Autodesk Inventor part; units mm, degrees
(part 2 of 2)
  spline S48 degree 3 poles (14.8423, 75.2854) (14.8523, 75.2852) (14.8732, 75.2847) (14.9051, 75.2815) (14.9386, 75.2762) (14.9736, 75.2689) (15.0103, 75.2594) (15.0484, 75.248) (15.0882, 75.2343) (15.115, 75.224) (15.1287, 75.2187) knots 0 0 0 0 0.102203 0.211023 0.3251 0.446502 0.573788 0.708901 0.850358 1 1 1 1
  line L109 (11.6821, 74.5687) -> (11.0654, 75.8687)
  line L110 (11.0654, 75.8687) -> (11.0487, 75.8687)
  line L111 (11.0487, 75.8687) -> (10.4487, 74.5687)
  line L112 (10.4487, 74.5687) -> (10.5756, 74.5687)
  line L113 (10.5756, 74.5687) -> (10.7677, 74.9854)
  line L114 (10.7677, 74.9854) -> (11.3571, 74.9854)
  line L115 (11.3571, 74.9854) -> (11.5547, 74.5687)
  line L116 (11.5547, 74.5687) -> (11.6821, 74.5687)
  spline S49 degree 3 poles (10.1721, 75.2263) (10.1715, 75.2497) (10.1703, 75.2957) (10.1607, 75.3632) (10.1452, 75.4279) (10.1231, 75.4896) (10.0951, 75.5487) (10.0606, 75.6047) (10.0198, 75.658) (9.9732, 75.7078) (9.9221, 75.7533) (9.8674, 75.7934) (9.8092, 75.8267) (9.7481, 75.8546) (9.6837, 75.876) (9.616, 75.891) (9.5453, 75.9003) (9.4971, 75.9015) (9.4726, 75.9021) knots 0 0 0 0 0.064558 0.127014 0.187955 0.248014 0.307748 0.368235 0.42947 0.492743 0.556258 0.618217 0.679655 0.741246 0.803415 0.866815 0.932328 1 1 1 1
  spline S50 degree 3 poles (9.4726, 75.9021) (9.4576, 75.9019) (9.4281, 75.9015) (9.3843, 75.8981) (9.3418, 75.8923) (9.3003, 75.8845) (9.2598, 75.8747) (9.2205, 75.8621) (9.1822, 75.8476) (9.1451, 75.8309) (9.1095, 75.8121) (9.0753, 75.7915) (9.0428, 75.7691) (9.0118, 75.7451) (8.9828, 75.719) (8.955, 75.6914) (8.9292, 75.6616) (8.9134, 75.6407) (8.9054, 75.6302) knots 0 0 0 0 0.068548 0.135683 0.201215 0.265682 0.329267 0.392395 0.45507 0.517127 0.57879 0.63974 0.700192 0.759806 0.819628 0.879355 0.939512 1 1 1 1
  line L117 (8.9054, 75.6302) -> (9.0075, 75.5521)
  spline S51 degree 3 poles (9.0075, 75.5521) (9.0148, 75.5607) (9.0292, 75.578) (9.0525, 75.6022) (9.0768, 75.6249) (9.102, 75.6461) (9.1286, 75.6652) (9.1561, 75.6832) (9.1847, 75.6992) (9.2244, 75.7187) (9.2763, 75.7391) (9.3416, 75.7561) (9.4097, 75.767) (9.4562, 75.7681) (9.4799, 75.7687) knots 0 0 0 0 0.063163 0.125475 0.187121 0.248294 0.309295 0.36985 0.430973 0.492456 0.616148 0.740844 0.868183 1 1 1 1
  spline S52 degree 3 poles (9.4799, 75.7687) (9.4929, 75.7686) (9.5188, 75.7683) (9.5573, 75.7643) (9.5951, 75.7588) (9.6322, 75.7506) (9.6684, 75.7402) (9.7041, 75.7278) (9.7387, 75.7124) (9.7727, 75.6954) (9.8054, 75.6763) (9.8362, 75.6554) (9.8652, 75.6329) (9.8923, 75.6089) (9.9176, 75.5834) (9.941, 75.5562) (9.9622, 75.5273) (9.9818, 75.4971) (9.9993, 75.4657) (10.014, 75.4329) (10.027, 75.3995) (10.0373, 75.3649) (10.0454, 75.3294) (10.0511, 75.2929) (10.0549, 75.2555) (10.0552, 75.2302) (10.0554, 75.2174) knots 0 0 0 0 0.043955 0.087502 0.130463 0.172752 0.215403 0.25765 0.300153 0.343121 0.385925 0.427686 0.468818 0.509492 0.549883 0.58998 0.630405 0.670869 0.711384 0.751627 0.791776 0.832459 0.873319 0.914543 0.956924 1 1 1 1
  spline S53 degree 3 poles (10.0554, 75.2174) (10.0549, 75.1982) (10.054, 75.1605) (10.0458, 75.1052) (10.0334, 75.0523) (10.0147, 75.002) (9.9917, 74.9538) (9.9627, 74.9084) (9.929, 74.8651) (9.8903, 74.8251) (9.8478, 74.7885) (9.8022, 74.7563) (9.7536, 74.7294) (9.7026, 74.707) (9.6487, 74.6899) (9.5921, 74.6778) (9.5329, 74.6699) (9.4924, 74.6691) (9.4718, 74.6687) knots 0 0 0 0 0.064323 0.12629 0.186726 0.246146 0.305576 0.365429 0.426326 0.48884 0.551725 0.613919 0.675484 0.737334 0.800229 0.864502 0.931041 1 1 1 1
  spline S54 degree 3 poles (9.4718, 74.6687) (9.4491, 74.6694) (9.4044, 74.6706) (9.3389, 74.6811) (9.2762, 74.698) (9.2163, 74.7217) (9.1593, 74.7526) (9.1053, 74.79) (9.054, 74.8343) (9.0232, 74.8681) (9.0075, 74.8854) knots 0 0 0 0 0.128515 0.252949 0.374755 0.49594 0.617181 0.740909 0.867811 1 1 1 1
  line L118 (9.0075, 74.8854) -> (8.9054, 74.8081)
  spline S55 degree 3 poles (8.9054, 74.8081) (8.9136, 74.7975) (8.93, 74.7763) (8.9565, 74.7465) (8.9845, 74.7184) (9.0141, 74.6924) (9.045, 74.6678) (9.0777, 74.6454) (9.1118, 74.6249) (9.1472, 74.6061) (9.1839, 74.5894) (9.2218, 74.5751) (9.2607, 74.5628) (9.3007, 74.5527) (9.3418, 74.5448) (9.3839, 74.5395) (9.4271, 74.5359) (9.4563, 74.5356) (9.471, 74.5354) knots 0 0 0 0 0.061674 0.123053 0.183475 0.243727 0.304279 0.364863 0.425946 0.487391 0.54922 0.611144 0.673529 0.736961 0.800785 0.866013 0.932101 1 1 1 1
  spline S56 degree 3 poles (9.471, 74.5354) (9.485, 74.5355) (9.5126, 74.5357) (9.5535, 74.5388) (9.5932, 74.5431) (9.6318, 74.5495) (9.6693, 74.557) (9.7056, 74.5671) (9.7408, 74.5785) (9.775, 74.5918) (9.8081, 74.6069) (9.84, 74.6239) (9.8706, 74.6427) (9.9004, 74.6629) (9.9289, 74.6852) (9.9562, 74.7092) (9.9827, 74.7349) (9.999, 74.7534) (10.0072, 74.7627) knots 0 0 0 0 0.069663 0.13775 0.203917 0.26878 0.332414 0.394754 0.45618 0.516996 0.577396 0.637198 0.696999 0.756756 0.816554 0.876948 0.938132 1 1 1 1
  spline S57 degree 3 poles (10.0072, 74.7627) (10.0204, 74.7789) (10.0465, 74.8111) (10.08, 74.8632) (10.1087, 74.9176) (10.1318, 74.9746) (10.15, 75.034) (10.1625, 75.0959) (10.1707, 75.1603) (10.1716, 75.204) (10.1721, 75.2263) knots 0 0 0 0 0.124329 0.247156 0.36878 0.490734 0.613614 0.738958 0.867311 1 1 1 1
  line L119 (7.0994, 75.8187) -> (7.3122, 75.8187)
  line L120 (7.4998, 74.7187) -> (7.0994, 75.8187)
  line L121 (6.9998, 74.7187) -> (7.4998, 74.7187)
  line L122 (6.5994, 75.8187) -> (6.9998, 74.7187)
  line L123 (6.3866, 75.8187) -> (6.5994, 75.8187)
  line L124 (6.7869, 74.7187) -> (6.3866, 75.8187)
  line L125 (6.5869, 74.7187) -> (6.7869, 74.7187)
  line L126 (6.6597, 74.5187) -> (6.5869, 74.7187)
  line L127 (7.7854, 74.5187) -> (6.6597, 74.5187)
  line L128 (7.3122, 75.8187) -> (7.7854, 74.5187)
  line L129 (12.4754, 74.5687) -> (12.4921, 74.5687)
  line L130 (12.4921, 74.5687) -> (13.0421, 75.8687)
  line L131 (13.0421, 75.8687) -> (12.9171, 75.8687)
  line L132 (12.9171, 75.8687) -> (12.4837, 74.8443)
  line L133 (12.4837, 74.8443) -> (12.0504, 75.8687)
  line L134 (12.0504, 75.8687) -> (11.9254, 75.8687)
  line L135 (11.9254, 75.8687) -> (12.4754, 74.5687)
  spline S58 degree 3 poles (13.2854, 75.2182) (13.2856, 75.1983) (13.2861, 75.1596) (13.2886, 75.1029) (13.2934, 75.0495) (13.2994, 74.999) (13.3077, 74.9518) (13.318, 74.9077) (13.3294, 74.8665) (13.3434, 74.8285) (13.3588, 74.7933) (13.3755, 74.7603) (13.3935, 74.7294) (13.413, 74.7008) (13.4338, 74.6743) (13.4564, 74.6504) (13.48, 74.6284) (13.5051, 74.6088) (13.5312, 74.5917) (13.5579, 74.5764) (13.5857, 74.5641) (13.6139, 74.5535) (13.6429, 74.5454) (13.6727, 74.5398) (13.7032, 74.5359) (13.7238, 74.5356) (13.7341, 74.5354) knots 0 0 0 0 0.065063 0.126773 0.185516 0.240765 0.29298 0.34225 0.388919 0.432776 0.474628 0.514775 0.553606 0.591426 0.628028 0.663804 0.698984 0.733591 0.767628 0.801208 0.834264 0.866981 0.89972 0.932702 0.966176 1 1 1 1
  spline S59 degree 3 poles (13.7341, 74.5354) (13.7443, 74.5356) (13.7646, 74.5359) (13.7945, 74.5394) (13.8236, 74.5451) (13.8519, 74.5531) (13.8797, 74.5628) (13.9065, 74.5755) (13.9326, 74.5901) (13.9579, 74.6068) (13.9821, 74.6258) (14.0051, 74.6469) (14.0266, 74.6705) (14.0465, 74.6963) (14.0654, 74.7241) (14.0828, 74.7541) (14.0989, 74.7864) (14.1137, 74.8211) (14.1267, 74.8586) (14.1382, 74.8995) (14.1473, 74.9442) (14.1551, 74.9921) (14.1614, 75.0436) (14.1657, 75.0987) (14.1684, 75.1573) (14.1686, 75.1976) (14.1687, 75.2182) knots 0 0 0 0 0.033787 0.066622 0.099285 0.131361 0.163585 0.196104 0.228902 0.262158 0.295991 0.330218 0.36506 0.400951 0.43762 0.475708 0.515381 0.556414 0.599765 0.646424 0.696431 0.749782 0.806573 0.867436 0.931887 1 1 1 1
  spline S60 degree 3 poles (14.1687, 75.2182) (14.1686, 75.239) (14.1684, 75.2795) (14.1657, 75.3385) (14.1614, 75.3938) (14.1554, 75.4455) (14.1481, 75.4936) (14.1383, 75.5378) (14.1273, 75.5786) (14.1144, 75.6159) (14.1, 75.6503) (14.0842, 75.6824) (14.0665, 75.7121) (14.048, 75.74) (14.0277, 75.7656) (14.0065, 75.7893) (13.9833, 75.8104) (13.959, 75.8297) (13.9333, 75.8466) (13.9071, 75.8614) (13.8801, 75.8741) (13.8522, 75.8841) (13.8237, 75.8924) (13.7945, 75.898) (13.7646, 75.9016) (13.7443, 75.9019) (13.7341, 75.9021) knots 0 0 0 0 0.068595 0.133246 0.194313 0.251279 0.304513 0.354235 0.400481 0.443411 0.484015 0.523252 0.561042 0.5979 0.633518 0.668314 0.702496 0.736685 0.770293 0.803437 0.835913 0.86846 0.900847 0.933467 0.966258 1 1 1 1
  spline S61 degree 3 poles (13.7341, 75.9021) (13.7238, 75.9019) (13.7032, 75.9015) (13.6728, 75.8981) (13.6431, 75.8923) (13.6142, 75.8842) (13.586, 75.8741) (13.5585, 75.8614) (13.5317, 75.8467) (13.5059, 75.8294) (13.481, 75.81) (13.4574, 75.7882) (13.4352, 75.7641) (13.4142, 75.7379) (13.3948, 75.7092) (13.3764, 75.6785) (13.3599, 75.6452) (13.3441, 75.6098) (13.3304, 75.5714) (13.318, 75.5303) (13.308, 75.4859) (13.2997, 75.4384) (13.2933, 75.3878) (13.2886, 75.334) (13.2861, 75.2771) (13.2856, 75.2382) (13.2854, 75.2182) knots 0 0 0 0 0.033788 0.067194 0.099862 0.132567 0.165151 0.197913 0.231319 0.265083 0.299255 0.334399 0.369943 0.406284 0.444064 0.482998 0.523354 0.565537 0.609613 0.656391 0.705885 0.758325 0.813832 0.872795 0.934722 1 1 1 1
  line L136 (19.4354, 75.2187) -> (19.3021, 75.8687)
  line L137 (19.3021, 75.8687) -> (18.7687, 75.8687)
  line L138 (18.7687, 75.8687) -> (18.7687, 75.7354)
  line L139 (18.7687, 75.7354) -> (19.2109, 75.7354)
  line L140 (19.2109, 75.7354) -> (19.281, 75.3935)
  spline S62 degree 3 poles (19.281, 75.3935) (19.2672, 75.3973) (19.2405, 75.4046) (19.2012, 75.4128) (19.1638, 75.4177) (19.1396, 75.4184) (19.1278, 75.4187) knots 0 0 0 0 0.275068 0.532901 0.773973 1 1 1 1
  spline S63 degree 3 poles (19.1278, 75.4187) (19.1133, 75.4184) (19.0848, 75.4178) (19.043, 75.4119) (19.0032, 75.4025) (18.9653, 75.3895) (18.9293, 75.3728) (18.8956, 75.352) (18.8636, 75.3276) (18.8339, 75.2996) (18.8069, 75.2688) (18.7832, 75.2357) (18.7631, 75.2006) (18.7469, 75.1632) (18.734, 75.1238) (18.7254, 75.0821) (18.7197, 75.0385) (18.7191, 75.0087) (18.7187, 74.9935) knots 0 0 0 0 0.065808 0.129394 0.190894 0.251281 0.310815 0.370371 0.430768 0.492881 0.555104 0.616067 0.677256 0.73826 0.800762 0.864778 0.931045 1 1 1 1
  spline S64 degree 3 poles (18.7187, 74.9935) (18.719, 74.9829) (18.7195, 74.9618) (18.722, 74.9306) (18.7268, 74.9) (18.7332, 74.8701) (18.7416, 74.8408) (18.7517, 74.8122) (18.7641, 74.7845) (18.7777, 74.7572) (18.7931, 74.7312) (18.8101, 74.7068) (18.828, 74.6837) (18.8474, 74.6622) (18.8682, 74.6424) (18.8904, 74.6243) (18.9137, 74.6074) (18.9384, 74.5925) (18.9641, 74.5787) (18.9911, 74.5675) (19.0187, 74.5574) (19.0475, 74.5494) (19.0772, 74.5431) (19.108, 74.5388) (19.1398, 74.5357) (19.1613, 74.5355) (19.1721, 74.5354) knots 0 0 0 0 0.044014 0.087434 0.130118 0.172554 0.214555 0.256298 0.298438 0.340849 0.382715 0.423924 0.464246 0.504074 0.543862 0.583567 0.623094 0.663229 0.703551 0.743938 0.784541 0.82575 0.867757 0.910745 0.954914 1 1 1 1
  spline S65 degree 3 poles (19.1721, 74.5354) (19.1851, 74.5357) (19.2106, 74.5362) (19.2479, 74.5414) (19.2838, 74.549) (19.318, 74.5604) (19.3509, 74.5746) (19.3818, 74.5927) (19.4118, 74.6131) (19.4395, 74.6372) (19.4651, 74.6635) (19.4881, 74.6921) (19.5086, 74.7225) (19.5262, 74.7547) (19.5413, 74.7889) (19.5531, 74.8249) (19.5626, 74.8628) (19.5667, 74.8888) (19.5687, 74.9021) knots 0 0 0 0 0.065421 0.128708 0.190236 0.250724 0.310637 0.370766 0.431615 0.493523 0.555883 0.617342 0.678668 0.740711 0.802985 0.866803 0.932347 1 1 1 1
  line L141 (19.5687, 74.9021) -> (19.4521, 74.9021)
  spline S66 degree 3 poles (19.4521, 74.9021) (19.4492, 74.8897) (19.4437, 74.8658) (19.4316, 74.8324) (19.4168, 74.8025) (19.3991, 74.7759) (19.3781, 74.7528) (19.3542, 74.7321) (19.3273, 74.7135) (19.2974, 74.6979) (19.2659, 74.6847) (19.233, 74.6759) (19.1994, 74.6697) (19.1767, 74.669) (19.1653, 74.6687) knots 0 0 0 0 0.094687 0.181994 0.264377 0.34218 0.418618 0.496509 0.577369 0.661511 0.746733 0.831258 0.915206 1 1 1 1
  spline S67 degree 3 poles (19.1653, 74.6687) (19.1542, 74.669) (19.1323, 74.6696) (19.1001, 74.6743) (19.0689, 74.6814) (19.0392, 74.692) (19.0104, 74.705) (18.9832, 74.7216) (18.9569, 74.7407) (18.9322, 74.7626) (18.9096, 74.7867) (18.8897, 74.8125) (18.873, 74.8401) (18.859, 74.8688) (18.8484, 74.8992) (18.8408, 74.9309) (18.8363, 74.9642) (18.8357, 74.9869) (18.8354, 74.9984) knots 0 0 0 0 0.064207 0.126425 0.18768 0.248216 0.308305 0.369661 0.431699 0.495947 0.559758 0.622295 0.683911 0.745092 0.80674 0.869087 0.93329 1 1 1 1
  spline S68 degree 3 poles (18.8354, 74.9984) (18.8356, 75.0088) (18.8361, 75.0293) (18.84, 75.0591) (18.8468, 75.0874) (18.8563, 75.1142) (18.8683, 75.1395) (18.8829, 75.1634) (18.9005, 75.1856) (18.9206, 75.2061) (18.9426, 75.225) (18.9669, 75.2411) (18.993, 75.2546) (19.0206, 75.2663) (19.0503, 75.2747) (19.0815, 75.281) (19.1147, 75.2846) (19.1373, 75.2851) (19.1489, 75.2854) knots 0 0 0 0 0.065351 0.127916 0.18836 0.247216 0.30563 0.36377 0.422661 0.482687 0.5433 0.604118 0.664965 0.727413 0.791468 0.858055 0.927037 1 1 1 1
  spline S69 degree 3 poles (19.1489, 75.2854) (19.159, 75.2852) (19.1798, 75.2847) (19.2117, 75.2815) (19.2453, 75.2762) (19.2803, 75.2689) (19.3169, 75.2594) (19.3551, 75.248) (19.3948, 75.2343) (19.4216, 75.224) (19.4354, 75.2187) knots 0 0 0 0 0.102203 0.211023 0.3251 0.446502 0.573788 0.708901 0.850358 1 1 1 1
  line L142 (0, 0) -> (0, 80)
  point P0 (43, 40)
  point P1 (7.7854, 7.6813)
  point P2 (7.7854, 72.3187)
  constraints: 284 end point, 140 symmetric about line, 60 point on circle, 36 horizontal, 34 centre point, 1 midpoint, 161 other
extrude "Выдавливание32" cut sketch "Эскиз43" against normal blind 5 contours A15 | A16 | A32 | A33
sketch "Эскиз45" plane through (10, 0, 0) normal (1, 0, 0) x (0, 0, -1)
  arc A0 (9.15, 62) -> (-9.15, 62) centre (0, 62) ccw projected
  circle A1 centre (0, 62) radius 11
  point P0 (0, 0)
  dimension "d165" = 22
  constraints: 1 centre point, 1 coincident
  measures "d165" diameter of A1
extrude "Выдавливание33" cut sketch "Эскиз45" against normal blind 10
sketch "Эскиз46" plane through (-43, 34, -40) normal (0, 1, 0) x (1, 0, 0)
  line L0 (10, -80) -> (0, -80) projected
  line L1 (0, -80) -> (15, -80)
  line L2 (15, -80) -> (15, -30)
  line L3 (15, -30) -> (0, -30)
  line L4 (0, -30) -> (0, -80)
  line L5 (15, -80) -> (15, -50)
  circle A0 centre (15, -50) radius 1.95
  circle A1 centre (15, -30) radius 1.95
  point P0 (43, -40)
  dimension "d168" = 15
  dimension "d169" = 50
  dimension "d170" = 30
  dimension "d171" = 3.9
  dimension "d172" = 3.9
  constraints: 10 end point, 2 centre point, 2 coincident, 2 parallel, 1 horizontal, 1 perpendicular, 1 point on line
  measures "d168" distance of L3.end L2.end
  measures "d169" distance of L2.end L1.end
  measures "d170" distance of L1.end L5.end
  measures "d171" diameter of A0
  measures "d172" diameter of A1
extrude "Выдавливание34" cut sketch "Эскиз46" against normal blind 10 contours A0 L2 | L2 A0 | A1 L2 L3 | L3 L2 A1
sketch "Эскиз47" plane through (5, 34, -28.9) normal (-1, 0, 0) x (0, 0, 1)
  arc A0 (38.9, 23.4174) -> (18.9, 23.4174) centre (28.9, 28) ccw projected
  line L0 (38.9, 23.4174) -> (38.9, 0) projected
  line L1 (57.8, 0) -> (38.9, 0) projected
  line L2 (57.8, 0) -> (57.8, 37.25) projected
  line L3 (55.05, 40) -> (57.8, 37.25) projected
  line L4 (2.75, 40) -> (55.05, 40) projected
  line L5 (0, 37.25) -> (2.75, 40) projected
  line L6 (0, 0) -> (0, 37.25) projected
  line L7 (18.9, 0) -> (0, 0) projected
  line L8 (18.9, 0) -> (18.9, 23.4174) projected
  circle A1 centre (42.4, 13.5) radius 1.3 projected
  circle A2 centre (15.4, 21.5) radius 1.3 projected
  circle A3 centre (15.4, 5.5) radius 1.3 projected
  circle A4 centre (15.4, 13.5) radius 1.3 projected
  circle A5 centre (42.4, 5.5) radius 1.3 projected
  circle A6 centre (42.4, 21.5) radius 1.3 projected
  point P0 (28.9, -34)
move faces "Перенос2" translate (0, 4, 0) faces at (6.6667, 74, -8.7167)
move faces "Перенос3" translate (0, -10, 0) faces at (8.2105, 24, -33.9873) (8.2105, 24, 34.9127)
equation "\"d3\" = d2"
equation "\"d5\" = d4"
equation "\"d6\" = d2"
equation "\"d7\" = d2"
equation "\"d9\" = d8"
equation "\"d10\" = d8"
equation "\"d11\" = d8"
equation "\"d17\" = d14"
equation "\"d18\" = d16"
equation "\"d19\" = d14"
equation "\"d21\" = d16"
equation "\"d22\" = d16"
equation "\"d23\" = d14"
